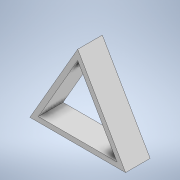
# Autodesk Inventor part: dishRing
Saved by Autodesk Inventor 2022.1 (Build 261234020, 234B)
## iProperties
Created: 2021-11-11
Part Number: dishRing
Material: Generic
Document SubType Name: Modeling
Designer: yiunf
Density: 1 g/cm^3
Appearance: Default
Author: yiunf
## iProperties of the stored document dishRing_3DPrint.ipt
Created: 2021-11-11
Part Number: dishRing_3DPrint
Material: Generic
Document SubType Name: Modeling
Designer: yiunf
Density: 1 g/cm^3
Appearance: Default
Author: yiunf
Autodesk Inventor part; units mm, degrees
ref_plane "YZ Plane" through (0, 0, 0) normal (1, 0, 0) x (0, 1, 0)
ref_plane "XZ Plane" through (0, 0, 0) normal (0, 1, 0) x (-1, 0, 0)
ref_plane "XY Plane" through (0, 0, 0) normal (0, 0, 1) x (1, 0, 0)
sketch "Sketch1" plane through (0, 0, 0) normal (0, 0, 1) x (1, 0, 0)
  line L0 (0, 0) -> (-16, 0)
  line L1 (-16, 0) -> (-8, 13.8564)
  line L2 (-8, 13.8564) -> (0, 0)
  line L3 (0, 0) -> (-16, 0)
  line L4 (-8, 15.8564) -> (-17.7321, -1)
  line L5 (-17.7321, -1) -> (1.7321, -1)
  line L6 (1.7321, -1) -> (-8, 15.8564)
  dimension "d4" = 16
  dimension "d5" = 1
  constraints: 14 end point, 2 coincident, 1 collinear, 1 horizontal, 2 other
  measures "d4" distance of L0.start L0.end
  measures "d5" distance between parallel lines of L1 L4
extrude "Extrusion1" add sketch "Sketch1" along normal blind 5
body "Solid1"
